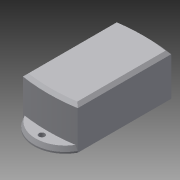
# Autodesk Inventor part: 12v_psu
Saved by Autodesk Inventor 2013 SP2 (Build 170200200, 200)
## iProperties
Created: 2018-11-12
Part Number: 12v_psu
Material: Generic
Document SubType Name: Modeling
Designer: alex
Density: 1 g/cm^3
Mass: 67.8406 g
Surface Area: 107.001 cm^2
Volume: 67.8406 cm^3
Author: alex
Autodesk Inventor part; units mm, degrees
ref_plane "YZ Plane" through (0, 0, 0) normal (1, 0, 0) x (0, 1, 0)
ref_plane "XZ Plane" through (0, 0, 0) normal (0, 1, 0) x (-1, 0, 0)
ref_plane "XY Plane" through (0, 0, 0) normal (0, 0, 1) x (1, 0, 0)
sketch "Sketch1" plane through (0, 0, 0) normal (0, 1, 0) x (-1, 0, 0)
  line L0 (18.5, 15.75) -> (-18.5, 15.75)
  line L1 (-18.5, 15.75) -> (-18.5, -15.75)
  line L2 (-18.5, -15.75) -> (18.5, -15.75)
  line L3 (18.5, -15.75) -> (18.5, 15.75)
  line L4 (18.5, 15.75) -> (-18.5, -15.75) construction
  line L5 (-18.5, 15.75) -> (18.5, -15.75) construction
  line L6 (0, -15.75) -> (0, -17.25)
  arc A0 (-18.5, -15.75) -> (18.5, -15.75) centre (0, 97.5833) ccw
  line L7 (-18.5, 15.75) -> (-18.5, 47.25)
  line L8 (-18.5, 47.25) -> (18.5, 47.25)
  line L9 (18.5, 47.25) -> (18.5, 15.75)
  line L10 (18.5, 15.75) -> (-18.5, 47.25) construction
  line L11 (-18.5, 15.75) -> (18.5, 47.25) construction
  line L12 (0, 47.25) -> (0, 48.75)
  arc A1 (18.5, 47.25) -> (-18.5, 47.25) centre (0, -66.0833) ccw
  point P0 (0, 0)
  point P1 (0, 31.5)
  dimension "d5" = 37
  dimension "d6" = 31.5
  dimension "d7" = 1.5
  constraints: 26 end point, 6 point on circle, 6 symmetric about line, 5 midpoint, 3 parallel, 2 centre point, 1 horizontal, 1 perpendicular, 1 other
  measures "d5" distance of L2.end L1.end
  measures "d6" distance of L1.end L0.end
  measures "d7" distance of L6.start L6.end
extrude "Extrusion1" add sketch "Sketch1" along normal blind 28
sketch "Sketch2" plane through (0, 0, 0) normal (0, -1, 0) x (1, 0, 0)
  arc A0 (-18.5, -15.75) -> (18.5, -15.75) centre (0, 97.5833) ccw projected
  line L0 (18.5, 47.25) -> (18.5, -15.75) projected
  line L1 (-18.5, -15.75) -> (-18.5, 47.25) projected
  line L2 (0, -17.25) -> (0, 58.25)
  arc A1 (18.5, 47.25) -> (-18.5, 47.25) centre (0, 37.1932) ccw
  point P0 (0, 0)
  dimension "d10" = 75.5
  constraints: 4 point on circle, 2 end point, 1 centre point, 1 parallel
  measures "d10" distance of L2.start L2.end
extrude "Extrusion2" add sketch "Sketch2" against normal blind 4
chamfer "Chamfer1" distance 2 angle 45 4 edges at (-18.5, 28, 15.75) (0, 28, 48.75) (0, 28, -17.25) (18.5, 28, 15.75)
chamfer "Chamfer2" distance 3 angle 20 1 edges at (0, 4, 58.25) measured on face at (13.1668, 2.6667, 53.6257)
sketch "Sketch3" plane through (0, 4, 0) normal (0, 1, 0) x (1, 0, 0)
  arc A0 (-17.1187, -47.4669) -> (17.1187, -47.4669) centre (0, -37.1932) ccw projected
  arc A1 (-17.1187, -47.4669) -> (17.1187, -47.4669) centre (0, 66.0833) ccw projected
  line L0 (0, -52.954) -> (0, -48.75)
  line L1 (0, -57.1581) -> (0, -52.954)
  point P0 (0, 0)
  constraints: 4 end point, 2 collinear, 2 point on circle
hole "Hole1" at (0, 4, 52.954) direction (0, -1, 0) diameter 4 end through all
body "Solid1"
